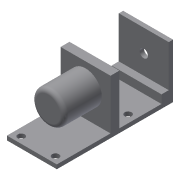
# Autodesk Inventor part: Motor Fixture
Saved by Autodesk Inventor 2015 (Build 190159000, 159)
## iProperties
Created: 2015-04-16
Part Number: Motor Fixture
Material: Generic
Document SubType Name: Modeling
Designer: jonathan
Density: 1 g/cm^3
Appearance: Default
Mass: 316.345 g
Surface Area: 670.541 cm^2
Volume: 316.345 cm^3
Author: jonathan
Autodesk Inventor part; units mm, degrees
ref_plane "YZ Plane" through (0, 0, 0) normal (1, 0, 0) x (0, 1, 0)
ref_plane "XZ Plane" through (0, 0, 0) normal (0, 1, 0) x (-1, 0, 0)
ref_plane "XY Plane" through (0, 0, 0) normal (0, 0, 1) x (1, 0, 0)
sketch "Sketch1" plane through (0, 0, 0) normal (0, 1, 0) x (-1, 0, 0)
  line L0 (-38.1, 88.708) -> (38.1, 88.708)
  line L1 (38.1, 88.708) -> (38.1, -88.708)
  line L2 (38.1, -88.708) -> (-38.1, -88.708)
  line L3 (-38.1, -88.708) -> (-38.1, 88.708)
  line L4 (-38.1, 88.708) -> (38.1, -88.708) construction
  line L5 (38.1, 88.708) -> (-38.1, -88.708) construction
  point P0 (0, 0)
  dimension "d0" = 76.2
  constraints: 12 end point, 2 midpoint, 2 parallel, 1 horizontal, 1 perpendicular
  measures "d0" distance of L0.start L0.end
extrude "Extrusion1" add sketch "Sketch1" along normal blind 6.35
sketch "Sketch2" plane through (0, 6.35, 0) normal (0, 1, 0) x (1, 0, 0)
  line L0 (38.1, -88.708) -> (38.1, 88.708) projected
  line L1 (-38.1, -6.787) -> (38.1, -6.787)
  line L2 (38.1, -6.787) -> (38.1, 6.787)
  line L3 (38.1, 6.787) -> (-38.1, 6.787)
  line L4 (-38.1, 6.787) -> (-38.1, -6.787)
  line L5 (-38.1, -6.787) -> (38.1, 6.787) construction
  line L6 (38.1, -6.787) -> (-38.1, 6.787) construction
  line L7 (-38.1, 88.708) -> (38.1, 88.708)
  line L8 (38.1, 88.708) -> (38.1, 82.0757)
  line L9 (38.1, 82.0757) -> (-38.1, 82.0757)
  line L10 (-38.1, 82.0757) -> (-38.1, 88.708)
  point P0 (0, 0)
  constraints: 20 end point, 4 parallel, 2 horizontal, 2 midpoint, 2 perpendicular, 1 point on line
extrude "Extrusion2" add sketch "Sketch2" along normal blind 76.2
sketch "Sketch3" plane through (0, 6.35, 0) normal (0, 1, 0) x (1, 0, 0)
  line L0 (-38.1, -88.708) -> (-38.1, 88.708) projected
  line L1 (38.1, 88.708) -> (-38.1, 88.708)
  line L2 (-38.1, 88.708) -> (-38.1, 70.9931)
  line L3 (-38.1, 70.9931) -> (38.1, 70.9931)
  line L4 (38.1, 70.9931) -> (38.1, 88.708)
  point P0 (0, 0)
  constraints: 8 end point, 2 parallel, 1 horizontal, 1 perpendicular, 1 point on line
extrude "Extrusion3" add sketch "Sketch3" along normal blind 12.7
sketch "Sketch4" plane through (-38.1, 6.35, 6.787) normal (0, 0, 1) x (1, 0, 0)
  circle A0 centre (38.1, 42.2042) radius 6.35
  point P0 (38.1, -6.35)
  dimension "d7" = 12.7
  constraints: 1 centre point
  measures "d7" diameter of A0
extrude "Extrusion4" cut sketch "Sketch4" against normal blind 100.0125
sketch "Sketch5" plane through (-38.1, 6.35, 6.787) normal (0, 0, 1) x (1, 0, 0)
  circle A0 centre (38.1, 42.2042) radius 24.7775
  circle A1 centre (38.1, 42.2042) radius 6.35 projected
  point P0 (38.1, -6.35)
  constraints: 1 centre point, 1 concentric
extrude "Extrusion5" add sketch "Sketch5" along normal blind 57.15 contours A0 | A1
fillet "Fillet1" radius 6.35 1 edges at (-24.7775, 48.5542, 63.937)
sketch "Sketch6" plane through (0, 6.35, 0) normal (0, 1, 0) x (1, 0, 0)
  circle A0 centre (-26.2107, -78.7534) radius 5.2502
  circle A1 centre (-26.2107, 31.9702) radius 5.2572
  point P0 (0, 0)
  constraints: 2 centre point
extrude "Extrusion6" cut sketch "Sketch6" against normal blind 25.4
mirror "Mirror1" about plane through (0, 0, 0) normal (1, 0, 0) of "Extrusion6"
sketch "Sketch7" plane through (38.1, 6.35, -6.787) normal (0, 0, -1) x (-1, 0, 0)
  circle A0 centre (22.9263, 42.0163) radius 3.3075
  point P0 (38.1, -6.35)
  constraints: 1 centre point
extrude "Extrusion7" cut sketch "Sketch7" against normal blind 25.4
mirror "Mirror2" about plane through (0, 0, 0) normal (1, 0, 0) of "Extrusion7"
sketch "Sketch8" plane through (0, 6.35, 0) normal (0, 1, 0) x (1, 0, 0)
  point P0 (0, 0)
body "Solid1"
